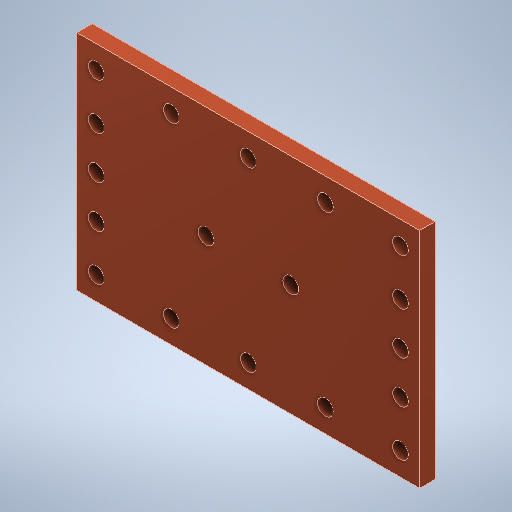
# Autodesk Inventor part: 1152
Saved by Autodesk Inventor 2025.1 (Build 291241000, 241)
## iProperties
Created: 2024-06-07
Part Number: 1152
Material: Kupfer
Document SubType Name: Modeling
Designer: ffogue
Density: 8.94 g/cm^3
Appearance: Kupfer - satiniert
Author: ffogue
Autodesk Inventor part; units mm, degrees
ref_plane "XZ Plane" through (0, 0, 0) normal (0, 1, 0) x (-1, 0, 0)
ref_plane "XY Plane" through (0, 0, 0) normal (0, 0, 1) x (1, 0, 0)
sketch "Skizze1" plane through (0, 0, 0) normal (0, 1, 0) x (-1, 0, 0)
  line L0 (0, 0) -> (-89, 0)
  line L1 (-89, 0) -> (-89, 58)
  line L2 (-89, 58) -> (0, 58)
  line L3 (0, 58) -> (0, 0)
  dimension "d0" = 58
  dimension "d1" = 89
  constraints: 8 end point, 2 parallel, 1 horizontal, 1 perpendicular
  measures "d0" distance between parallel lines of L0 L2
  measures "d1" distance between parallel lines of L1 L3
extrude "Extrusion1" add sketch "Skizze1" along normal blind 4
sketch "Skizze2" plane through (0, 4, 0) normal (0, 1, 0) x (1, 0, 0)
  line L0 (89, 0) -> (0, 0) projected
  line L1 (89, -58) -> (89, 0) projected
  line L2 (0, 0) -> (0, -58) projected
  line L3 (0, -58) -> (89, -58) projected
  point P0 (84, -6)
  point P1 (84, -52)
  point P2 (84, -40)
  point P3 (84, -18)
  point P4 (89, -29)
  point P5 (89, -29)
  dimension "d5" = 5
  dimension "d12" = 6
  dimension "d13" = 6
  dimension "d17" = 11
  dimension "d18" = 11
  constraints: 3 vertical alignment, 2 midpoint
  measures "d5" distance from line of point (84, -6) L1
  measures "d12" distance from line of L0 point (84, -6)
  measures "d13" distance from line of point (84, -52) L3
  measures "d17" vertical distance of point (89, -29) point (84, -40)
  measures "d18" vertical distance of point (84, -18) point (89, -29)
hole "Bohrung1" at (84, 4, 6) at (84, 4, 52) at (84, 4, 40) at (84, 4, 18) direction (0, -1, 0) diameter 4 depth 4
ref_plane "Arbeitsebene1" through (44.5, 0, 0) normal (1, 0, 0) x (0, 1, 0)
mirror "Spiegeln1" about plane through (44.5, 0, 0) normal (1, 0, 0) of "Bohrung1"
sketch "Skizze3" plane through (0, 4, 0) normal (0, 1, 0) x (1, 0, 0)
  line L0 (0, -58) -> (89, -58) projected
  circle A0 centre (84, -6) radius 2 projected
  line L1 (89, 0) -> (0, 0) projected
  point P0 (64.5, -6)
  point P1 (24.5, -6)
  point P2 (44.5, -6)
  point P3 (44.5, -58)
  point P4 (64.5, -52)
  point P5 (44.5, -52)
  point P6 (24.5, -52)
  dimension "d27" = 20
  dimension "d28" = 20
  dimension "d44" = 6
  dimension "d45" = 6
  constraints: 4 horizontal alignment, 4 vertical alignment, 1 midpoint
  measures "d27" distance of point (44.5, -6) point (64.5, -6)
  measures "d28" distance of point (24.5, -6) point (44.5, -6)
  measures "d44" distance from line of L1 point (64.5, -6)
  measures "d45" distance from line of L0 point (64.5, -52)
hole "Bohrung2" at (64.5, 4, 6) at (24.5, 4, 6) at (44.5, 4, 6) at (64.5, 4, 52) at (44.5, 4, 52) at (24.5, 4, 52) direction (0, -1, 0) diameter 4 depth 4
sketch "Skizze4" plane through (0, 0, 0) normal (0, -1, 0) x (1, 0, 0)
  line L0 (0, 0) -> (0, 58) projected
  circle A0 centre (5, 52) radius 2 projected
  circle A1 centre (84, 52) radius 2 projected
  point P0 (5, 29)
  point P1 (84, 29)
  point P2 (0, 29)
  constraints: 2 horizontal alignment, 2 vertical alignment, 1 midpoint
hole "Bohrung3" at (5, 0, 29) at (84, 0, 29) direction (0, 1, 0) diameter 4 end through all
sketch "Sketch9" plane through (0, 0, 0) normal (0, -1, 0) x (1, 0, 0)
  line L0 (0, 0) -> (0, 58) projected
  line L1 (0, 58) -> (89, 58) projected
  point P0 (33.5, 29)
  point P1 (55.5, 29)
  point P2 (0, 29)
  point P3 (44.5, 58)
  dimension "d67" = 22
  dimension "d68" = 11
  constraints: 2 horizontal alignment, 2 midpoint
  measures "d67" distance of point (55.5, 29) point (33.5, 29)
  measures "d68" horizontal distance of point (44.5, 58) point (33.5, 29)
hole "Hole4" at (55.5, 0, 29) at (33.5, 0, 29) direction (0, 1, 0) diameter 4 depth 4
